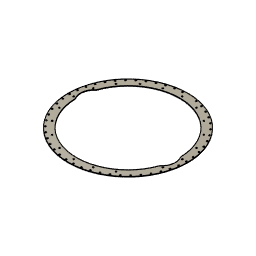
chopper_wheel v9 (Autodesk Fusion 360 design; units mm, degrees)
Autodesk Fusion 360 part; units mm, degrees
sketch "Sketch1" plane through (0, 0, 0) normal (0, 0, 1) x (1, 0, 0)
  circle A0 centre (0, 0) radius 190
  circle A1 centre (0, 0) radius 210
  dimension "d1" = 380
  dimension "d2" = 420
  constraint coincident A0.centre A1.centre
  constraint concentric A0 A1
  measures "d1" diameter of A0
  measures "d2" diameter of A1
extrude "Extrude1" add sketch "Sketch1" along normal blind 2
sketch "Sketch2" plane through (0, 0, 2) normal (0, 0, 1) x (-1, 0, 0)
  circle A0 centre (0, 0) radius 190
  circle A1 centre (0, 0) radius 210
  line L0 (200, 0) -> (190.2113, 61.8034)
  line L1 (190.2113, 61.8034) -> (161.8034, 117.5571)
  line L2 (161.8034, 117.5571) -> (117.5571, 161.8034)
  line L3 (117.5571, 161.8034) -> (61.8034, 190.2113)
  line L4 (61.8034, 190.2113) -> (0, 200)
  line L5 (0, 200) -> (-61.8034, 190.2113)
  line L6 (-61.8034, 190.2113) -> (-117.5571, 161.8034)
  line L7 (-117.5571, 161.8034) -> (-161.8034, 117.5571)
  line L8 (-161.8034, 117.5571) -> (-190.2113, 61.8034)
  line L9 (-190.2113, 61.8034) -> (-200, 0)
  line L10 (-200, 0) -> (-190.2113, -61.8034)
  line L11 (-190.2113, -61.8034) -> (-161.8034, -117.5571)
  line L12 (-161.8034, -117.5571) -> (-117.5571, -161.8034)
  line L13 (-117.5571, -161.8034) -> (-61.8034, -190.2113)
  line L14 (-61.8034, -190.2113) -> (0, -200)
  line L15 (0, -200) -> (61.8034, -190.2113)
  line L16 (61.8034, -190.2113) -> (117.5571, -161.8034)
  line L17 (117.5571, -161.8034) -> (161.8034, -117.5571)
  line L18 (161.8034, -117.5571) -> (190.2113, -61.8034)
  line L19 (190.2113, -61.8034) -> (200, 0)
  constraint coincident A0.centre A1.centre
hole "Hole1" at (-200, 0, 2) at (-190.2113, 61.8034, 2) at (-161.8034, 117.5571, 2) at (-117.5571, 161.8034, 2) at (-61.8034, 190.2113, 2) at (0, 200, 2) at (61.8034, 190.2113, 2) at (117.5571, 161.8034, 2) at (161.8034, 117.5571, 2) at (190.2113, 61.8034, 2) at (200, 0, 2) at (190.2113, -61.8034, 2) at (117.5571, -161.8034, 2) at (61.8034, -190.2113, 2) at (0, -200, 2) at (-61.8034, -190.2113, 2) at (-117.5571, -161.8034, 2) at (-161.8034, -117.5571, 2) at (-190.2113, -61.8034, 2) direction (0, 0, -1) diameter 4.5 depth 20 tip angle 180
sketch "Sketch3" plane through (0, 0, 2) normal (0, 0, 1) x (-1, 0, 0)
  circle A0 centre (161.8034, 117.5571) radius 2.25
  circle A1 centre (61.8034, 190.2113) radius 2.25
  circle A2 centre (-61.8034, 190.2113) radius 2.25
  circle A3 centre (-190.2113, 61.8034) radius 2.25
  circle A4 centre (-190.2113, -61.8034) radius 2.25
  circle A5 centre (-117.5571, -161.8034) radius 2.25
  circle A6 centre (0, -200) radius 2.25
  circle A7 centre (117.5571, -161.8034) radius 2.25
  circle A8 centre (190.2113, -61.8034) radius 2.25
  circle A9 centre (200, 0) radius 2.25
  circle A10 centre (161.8034, -117.5571) radius 2.25
  circle A11 centre (61.8034, -190.2113) radius 2.25
  circle A12 centre (-61.8034, -190.2113) radius 2.25
  circle A13 centre (-161.8034, -117.5571) radius 2.25
  circle A14 centre (-200, 0) radius 2.25
  circle A15 centre (-117.5571, 161.8034) radius 2.25
  circle A16 centre (0, 200) radius 2.25
  circle A17 centre (117.5571, 161.8034) radius 2.25
  circle A18 centre (190.2113, 61.8034) radius 2.25
  circle A19 centre (0, 0) radius 190
  circle A20 centre (0, 0) radius 210
  circle A21 centre (0, 0) radius 200
  line L0 (0, 0) -> (190.2113, -61.8034)
  line L1 (0, 0) -> (200, 0)
  line L2 (0, 0) -> (197.5377, -31.2869)
  line L3 (197.5377, -31.2869) -> (148.1533, -23.4652)
  circle A22 centre (148.1533, -23.4652) radius 50
  line L4 (197.5377, -31.2869) -> (-197.5377, 31.2869)
  line L5 (-197.5377, 31.2869) -> (-148.1533, 23.4652)
  circle A23 centre (-148.1533, 23.4652) radius 50
  dimension "d8" = 171
  dimension "d9" = 50
  dimension "d10" = 100
  dimension "d11" = 50
  dimension "d12" = 100
  constraint coincident A19.centre A20.centre
  constraint coincident A9.centre A21
  constraint coincident A8.centre L0.end
  constraint coincident A9.centre L1.end
  constraint parallel L2 L3
  constraint coincident L3.end A22.centre
  constraint coincident A21 L4.end
  constraint parallel L2 L4
  constraint coincident L4 L5.end
  constraint coincident L5.end A23.centre
  measures "d8" angle of L1 L2
  measures "d9" distance of L2.end L3.end
  measures "d10" diameter of A22
  measures "d11" distance of L4.end L5.end
  measures "d12" diameter of A23
extrude "Extrude2" cut sketch "Sketch3" against normal blind 2 contours A19 L1 L2 L3 A22 L4 | A19 L1 A22 | A19 L0 L2 L3 A22 L4 | A19 L0 A22 | A19 L4 L5 A23 | A19 L4 L5 A23 picked at (191.5682, -25.2216) picked at (191.2896, 0.4483) picked at (189.8761, -35.6021) picked at (181.7887, -59.5381) picked at (-189.6936, 36.3263) picked at (-191.6348, 24.0702)
sketch "Sketch4" plane through (0, 0, 2) normal (0, 0, 1) x (-1, 0, 0)
  arc A0 (179.4368, -62.4695) -> (189.9587, 3.9631) centre (148.1533, -23.4652) ccw
  arc A1 (-189.9587, -3.9631) -> (179.4368, -62.4695) centre (0, 0) ccw
  arc A2 (-179.4368, 62.4695) -> (-189.9587, -3.9631) centre (-148.1533, 23.4652) ccw
  arc A3 (189.9587, 3.9631) -> (-179.4368, 62.4695) centre (0, 0) ccw
  circle A4 centre (161.8034, 117.5571) radius 2.25
  circle A5 centre (61.8034, 190.2113) radius 2.25
  circle A6 centre (-61.8034, 190.2113) radius 2.25
  circle A7 centre (-190.2113, 61.8034) radius 2.25
  circle A8 centre (-190.2113, -61.8034) radius 2.25
  circle A9 centre (-117.5571, -161.8034) radius 2.25
  circle A10 centre (0, -200) radius 2.25
  circle A11 centre (117.5571, -161.8034) radius 2.25
  circle A12 centre (190.2113, -61.8034) radius 2.25
  circle A13 centre (200, 0) radius 2.25
  circle A14 centre (161.8034, -117.5571) radius 2.25
  circle A15 centre (61.8034, -190.2113) radius 2.25
  circle A16 centre (-61.8034, -190.2113) radius 2.25
  circle A17 centre (-161.8034, -117.5571) radius 2.25
  circle A18 centre (-200, 0) radius 2.25
  circle A19 centre (-117.5571, 161.8034) radius 2.25
  circle A20 centre (0, 200) radius 2.25
  circle A21 centre (117.5571, 161.8034) radius 2.25
  circle A22 centre (190.2113, 61.8034) radius 2.25
sketch "Sketch5" plane through (0, 0, 2) normal (0, 0, 1) x (-1, 0, 0)
  circle A0 centre (0, 0) radius 210
  circle A1 centre (0, 0) radius 220
  line L0 (-215, 0) -> (-213.3047, -26.9466)
  line L1 (-213.3047, -26.9466) -> (-208.2454, -53.4683)
  line L2 (-208.2454, -53.4683) -> (-199.9019, -79.1468)
  line L3 (-199.9019, -79.1468) -> (-188.4059, -103.577)
  line L4 (-188.4059, -103.577) -> (-173.9387, -126.3738)
  line L5 (-173.9387, -126.3738) -> (-156.7283, -147.1776)
  line L6 (-156.7283, -147.1776) -> (-137.0462, -165.6603)
  line L7 (-137.0462, -165.6603) -> (-115.2028, -181.5305)
  line L8 (-115.2028, -181.5305) -> (-91.5425, -194.5378)
  line L9 (-91.5425, -194.5378) -> (-66.4387, -204.4772)
  line L10 (-66.4387, -204.4772) -> (-40.287, -211.1918)
  line L11 (-40.287, -211.1918) -> (-13.5, -214.5757)
  line L12 (-13.5, -214.5757) -> (13.5, -214.5757)
  line L13 (13.5, -214.5757) -> (40.287, -211.1918)
  line L14 (40.287, -211.1918) -> (66.4387, -204.4772)
  line L15 (66.4387, -204.4772) -> (91.5425, -194.5378)
  line L16 (91.5425, -194.5378) -> (115.2028, -181.5305)
  line L17 (115.2028, -181.5305) -> (137.0462, -165.6603)
  line L18 (137.0462, -165.6603) -> (156.7283, -147.1776)
  line L19 (156.7283, -147.1776) -> (173.9387, -126.3738)
  line L20 (173.9387, -126.3738) -> (188.4059, -103.577)
  line L21 (188.4059, -103.577) -> (199.9019, -79.1468)
  line L22 (199.9019, -79.1468) -> (208.2454, -53.4683)
  line L23 (208.2454, -53.4683) -> (213.3047, -26.9466)
  line L24 (213.3047, -26.9466) -> (215, 0)
  line L25 (215, 0) -> (213.3047, 26.9466)
  line L26 (213.3047, 26.9466) -> (208.2454, 53.4683)
  line L27 (208.2454, 53.4683) -> (199.9019, 79.1468)
  line L28 (199.9019, 79.1468) -> (188.4059, 103.577)
  line L29 (188.4059, 103.577) -> (173.9387, 126.3738)
  line L30 (173.9387, 126.3738) -> (156.7283, 147.1776)
  line L31 (156.7283, 147.1776) -> (137.0462, 165.6603)
  line L32 (137.0462, 165.6603) -> (115.2028, 181.5305)
  line L33 (115.2028, 181.5305) -> (91.5425, 194.5378)
  line L34 (91.5425, 194.5378) -> (66.4387, 204.4772)
  line L35 (66.4387, 204.4772) -> (40.287, 211.1918)
  line L36 (40.287, 211.1918) -> (13.5, 214.5757)
  line L37 (13.5, 214.5757) -> (-13.5, 214.5757)
  line L38 (-13.5, 214.5757) -> (-40.287, 211.1918)
  line L39 (-40.287, 211.1918) -> (-66.4387, 204.4772)
  line L40 (-66.4387, 204.4772) -> (-91.5425, 194.5378)
  line L41 (-91.5425, 194.5378) -> (-115.2028, 181.5305)
  line L42 (-115.2028, 181.5305) -> (-137.0462, 165.6603)
  line L43 (-137.0462, 165.6603) -> (-156.7283, 147.1776)
  line L44 (-156.7283, 147.1776) -> (-173.9387, 126.3738)
  line L45 (-173.9387, 126.3738) -> (-188.4059, 103.577)
  line L46 (-188.4059, 103.577) -> (-199.9019, 79.1468)
  line L47 (-199.9019, 79.1468) -> (-208.2454, 53.4683)
  line L48 (-208.2454, 53.4683) -> (-213.3047, 26.9466)
  line L49 (-213.3047, 26.9466) -> (-215, 0)
  circle A2 centre (-215, 0) radius 2.5
  circle A3 centre (-213.3047, 26.9466) radius 2.5
  circle A4 centre (-208.2454, 53.4683) radius 2.5
  circle A5 centre (-199.9019, 79.1468) radius 2.5
  circle A6 centre (-188.4059, 103.577) radius 2.5
  circle A7 centre (-173.9387, 126.3738) radius 2.5
  circle A8 centre (-156.7283, 147.1776) radius 2.5
  circle A9 centre (-137.0462, 165.6603) radius 2.5
  circle A10 centre (-115.2028, 181.5305) radius 2.5
  circle A11 centre (-91.5425, 194.5378) radius 2.5
  circle A12 centre (-66.4387, 204.4772) radius 2.5
  circle A13 centre (-40.287, 211.1918) radius 2.5
  circle A14 centre (-13.5, 214.5757) radius 2.5
  circle A15 centre (13.5, 214.5757) radius 2.5
  circle A16 centre (40.287, 211.1918) radius 2.5
  circle A17 centre (66.4387, 204.4772) radius 2.5
  circle A18 centre (91.5425, 194.5378) radius 2.5
  circle A19 centre (115.2028, 181.5305) radius 2.5
  circle A20 centre (137.0462, 165.6603) radius 2.5
  circle A21 centre (156.7283, 147.1776) radius 2.5
  circle A22 centre (173.9387, 126.3738) radius 2.5
  circle A23 centre (188.4059, 103.577) radius 2.5
  circle A24 centre (199.9019, 79.1468) radius 2.5
  circle A25 centre (208.2454, 53.4683) radius 2.5
  circle A26 centre (213.3047, 26.9466) radius 2.5
  circle A27 centre (215, 0) radius 2.5
  circle A28 centre (213.3047, -26.9466) radius 2.5
  circle A29 centre (208.2454, -53.4683) radius 2.5
  circle A30 centre (199.9019, -79.1468) radius 2.5
  circle A31 centre (188.4059, -103.577) radius 2.5
  circle A32 centre (173.9387, -126.3738) radius 2.5
  circle A33 centre (156.7283, -147.1776) radius 2.5
  circle A34 centre (137.0462, -165.6603) radius 2.5
  circle A35 centre (115.2028, -181.5305) radius 2.5
  circle A36 centre (91.5425, -194.5378) radius 2.5
  circle A37 centre (66.4387, -204.4772) radius 2.5
  circle A38 centre (40.287, -211.1918) radius 2.5
  circle A39 centre (13.5, -214.5757) radius 2.5
  circle A40 centre (-13.5, -214.5757) radius 2.5
  circle A41 centre (-40.287, -211.1918) radius 2.5
  circle A42 centre (-66.4387, -204.4772) radius 2.5
  circle A43 centre (-91.5425, -194.5378) radius 2.5
  circle A44 centre (-115.2028, -181.5305) radius 2.5
  circle A45 centre (-137.0462, -165.6603) radius 2.5
  circle A46 centre (-156.7283, -147.1776) radius 2.5
  circle A47 centre (-173.9387, -126.3738) radius 2.5
  circle A48 centre (-188.4059, -103.577) radius 2.5
  circle A49 centre (-213.3047, -26.9466) radius 2.5
  circle A50 centre (-208.2454, -53.4683) radius 2.5
  circle A51 centre (-199.9019, -79.1468) radius 2.5
  dimension "d15" = 420
  dimension "d16" = 440
  dimension "d17" = 215
  dimension "d18" = 5
  dimension "d19" = 5
  dimension "d20" = 5
  dimension "d21" = 5
  dimension "d22" = 5
  dimension "d23" = 5
  dimension "d24" = 5
  dimension "d25" = 5
  dimension "d26" = 5
  dimension "d27" = 5
  dimension "d28" = 5
  dimension "d29" = 5
  dimension "d30" = 5
  dimension "d31" = 5
  dimension "d32" = 5
  dimension "d33" = 5
  dimension "d34" = 5
  dimension "d35" = 5
  dimension "d36" = 5
  dimension "d37" = 5
  dimension "d38" = 5
  dimension "d39" = 5
  dimension "d40" = 5
  dimension "d41" = 5
  dimension "d42" = 5
  dimension "d43" = 5
  dimension "d44" = 5
  dimension "d45" = 5
  dimension "d46" = 5
  dimension "d47" = 5
  dimension "d48" = 5
  dimension "d49" = 5
  dimension "d50" = 5
  dimension "d51" = 5
  dimension "d52" = 5
  dimension "d53" = 5
  dimension "d54" = 5
  dimension "d55" = 5
  dimension "d56" = 5
  dimension "d57" = 5
  dimension "d58" = 5
  dimension "d59" = 5
  dimension "d60" = 5
  dimension "d61" = 5
  dimension "d62" = 5
  dimension "d63" = 5
  dimension "d64" = 5
  dimension "d65" = 5
  dimension "d66" = 5
  dimension "d67" = 5
  constraint coincident A0.centre A1.centre
  constraint concentric A0 A1
  constraint coincident L0.start L49.end
  constraint coincident L48.end L49.start
  constraint coincident L47.end L48.start
  constraint coincident L46.end L47.start
  constraint coincident L45.end L46.start
  constraint coincident L44.end L45.start
  constraint coincident L43.end L44.start
  constraint coincident L42.end L43.start
  constraint coincident L41.end L42.start
  constraint coincident L40.end L41.start
  constraint coincident L39.end L40.start
  constraint coincident L38.end L39.start
  constraint coincident L37.end L38.start
  constraint coincident L36.end L37.start
  constraint coincident L35.end L36.start
  constraint coincident L34.end L35.start
  constraint coincident L33.end L34.start
  constraint coincident L32.end L33.start
  constraint coincident L31.end L32.start
  constraint coincident L30.end L31.start
  constraint coincident L29.end L30.start
  constraint coincident L28.end L29.start
  constraint coincident L27.end L28.start
  constraint coincident L26.end L27.start
  constraint coincident L25.end L26.start
  constraint coincident L24.end L25.start
  constraint coincident L23.end L24.start
  constraint coincident L22.end L23.start
  constraint coincident L21.end L22.start
  constraint coincident L20.end L21.start
  constraint coincident L19.end L20.start
  constraint coincident L18.end L19.start
  constraint coincident L17.end L18.start
  constraint coincident L16.end L17.start
  constraint coincident L15.end L16.start
  constraint coincident L14.end L15.start
  constraint coincident L13.end L14.start
  constraint coincident L12.end L13.start
  constraint coincident L11.end L12.start
  constraint coincident L10.end L11.start
  constraint coincident L9.end L10.start
  constraint coincident L8.end L9.start
  constraint coincident L7.end L8.start
  constraint coincident L6.end L7.start
  constraint coincident L5.end L6.start
  constraint coincident L4.end L5.start
  constraint coincident L3.end L4.start
  constraint coincident L0.end L1.start
  constraint coincident L1.end L2.start
  constraint coincident L2.end L3.start
  measures "d15" diameter of A0
  measures "d16" diameter of A1
  measures "d17" distance of L0.start A0.centre
  measures "d18" diameter of A2
  measures "d19" diameter of A3
  measures "d20" diameter of A4
  measures "d21" diameter of A5
  measures "d22" diameter of A6
  measures "d23" diameter of A7
  measures "d24" diameter of A8
  measures "d25" diameter of A9
  measures "d26" diameter of A10
  measures "d27" diameter of A11
  measures "d28" diameter of A12
  measures "d29" diameter of A13
  measures "d30" diameter of A14
  measures "d31" diameter of A15
  measures "d32" diameter of A16
  measures "d33" diameter of A17
  measures "d34" diameter of A18
  measures "d35" diameter of A19
  measures "d36" diameter of A20
  measures "d37" diameter of A21
  measures "d38" diameter of A22
  measures "d39" diameter of A23
  measures "d40" diameter of A24
  measures "d41" diameter of A25
  measures "d42" diameter of A26
  measures "d43" diameter of A27
  measures "d44" diameter of A28
  measures "d45" diameter of A29
  measures "d46" diameter of A30
  measures "d47" diameter of A31
  measures "d48" diameter of A32
  measures "d49" diameter of A33
  measures "d50" diameter of A34
  measures "d51" diameter of A35
  measures "d52" diameter of A36
  measures "d53" diameter of A37
  measures "d54" diameter of A38
  measures "d55" diameter of A39
  measures "d56" diameter of A40
  measures "d57" diameter of A41
  measures "d58" diameter of A42
  measures "d59" diameter of A43
  measures "d60" diameter of A44
  measures "d61" diameter of A45
  measures "d62" diameter of A46
  measures "d63" diameter of A47
  measures "d64" diameter of A48
  measures "d65" diameter of A49
  measures "d66" diameter of A50
  measures "d67" diameter of A51
extrude "Extrude3" add sketch "Sketch5" against normal blind 2 contours A1 | L0 L1 L2 L3 L4 L5 L6 L7 L8 L9 L10 L11 L12 L13 L14 L15 L16 L17 L18 L19 L20 L21 L22 L23 L24 L25 L26 L27 L28 L29 L30 L31 L32 L33 L34 L35 L36 L37 L38 L39 L40 L41 L42 L43 L44 L45 L46 L47 L48 L49 A2 A3 A4 A5 A6 A7 A8 A9 A10 A11 A12 A13 A14 A15 A16 A17 A18 A19 A20 A21 A22 A23 A24 A25 A26 A27 A28 A29 A30 A31 A32 A33 A34 A35 A36 A37 A38 A39 A40 A41 A42 A43 A44 A45 A46 A47 A48 A49 A50 A51
sketch "Sketch6" plane through (0, 0, 2) normal (0, 0, 1) x (-1, 0, 0)
  circle A0 centre (0, 0) radius 220
  circle A1 centre (188.4059, 103.577) radius 2.5
  circle A2 centre (-137.0462, 165.6603) radius 2.5
  circle A3 centre (91.5425, 194.5378) radius 2.5
  circle A4 centre (-66.4387, 204.4772) radius 2.5
  circle A5 centre (66.4387, 204.4772) radius 2.5
  circle A6 centre (173.9387, 126.3738) radius 2.5
  circle A7 centre (115.2028, -181.5305) radius 2.5
  circle A8 centre (199.9019, -79.1468) radius 2.5
  circle A9 centre (40.287, -211.1918) radius 2.5
  circle A10 centre (156.7283, 147.1776) radius 2.5
  circle A11 centre (-13.5, 214.5757) radius 2.5
  circle A12 centre (-40.287, 211.1918) radius 2.5
  circle A13 centre (137.0462, 165.6603) radius 2.5
  circle A14 centre (213.3047, -26.9466) radius 2.5
  circle A15 centre (213.3047, 26.9466) radius 2.5
  circle A16 centre (215, 0) radius 2.5
  circle A17 centre (208.2454, -53.4683) radius 2.5
  circle A18 centre (13.5, 214.5757) radius 2.5
  circle A19 centre (156.7283, -147.1776) radius 2.5
  circle A20 centre (115.2028, 181.5305) radius 2.5
  circle A21 centre (91.5425, -194.5378) radius 2.5
  circle A22 centre (199.9019, 79.1468) radius 2.5
  circle A23 centre (66.4387, -204.4772) radius 2.5
  circle A24 centre (137.0462, -165.6603) radius 2.5
  circle A25 centre (-115.2028, 181.5305) radius 2.5
  circle A26 centre (173.9387, -126.3738) radius 2.5
  circle A27 centre (-91.5425, 194.5378) radius 2.5
  circle A28 centre (208.2454, 53.4683) radius 2.5
  circle A29 centre (188.4059, -103.577) radius 2.5
  circle A30 centre (40.287, 211.1918) radius 2.5
  circle A31 centre (-13.5, -214.5757) radius 2.5
  circle A32 centre (-91.5425, -194.5378) radius 2.5
  circle A33 centre (-173.9387, 126.3738) radius 2.5
  circle A34 centre (-188.4059, 103.577) radius 2.5
  circle A35 centre (-199.9019, 79.1468) radius 2.5
  circle A36 centre (-208.2454, 53.4683) radius 2.5
  circle A37 centre (-213.3047, 26.9466) radius 2.5
  circle A38 centre (-215, 0) radius 2.5
  circle A39 centre (-213.3047, -26.9466) radius 2.5
  circle A40 centre (-208.2454, -53.4683) radius 2.5
  circle A41 centre (-199.9019, -79.1468) radius 2.5
  circle A42 centre (-188.4059, -103.577) radius 2.5
  circle A43 centre (-173.9387, -126.3738) radius 2.5
  circle A44 centre (-156.7283, -147.1776) radius 2.5
  circle A45 centre (-137.0462, -165.6603) radius 2.5
  circle A46 centre (-115.2028, -181.5305) radius 2.5
  circle A47 centre (-40.287, -211.1918) radius 2.5
  circle A48 centre (13.5, -214.5757) radius 2.5
  circle A49 centre (-66.4387, -204.4772) radius 2.5
  circle A50 centre (-156.7283, 147.1776) radius 2.5
  arc A51 (179.4368, -62.4695) -> (189.9587, 3.9631) centre (148.1533, -23.4652) ccw
  arc A52 (-189.9587, -3.9631) -> (179.4368, -62.4695) centre (0, 0) ccw
  arc A53 (-179.4368, 62.4695) -> (-189.9587, -3.9631) centre (-148.1533, 23.4652) ccw
  arc A54 (189.9587, 3.9631) -> (-179.4368, 62.4695) centre (0, 0) ccw
  circle A55 centre (161.8034, 117.5571) radius 2.25
  circle A56 centre (61.8034, 190.2113) radius 2.25
  circle A57 centre (-61.8034, 190.2113) radius 2.25
  circle A58 centre (-190.2113, 61.8034) radius 2.25
  circle A59 centre (-190.2113, -61.8034) radius 2.25
  circle A60 centre (-117.5571, -161.8034) radius 2.25
  circle A61 centre (0, -200) radius 2.25
  circle A62 centre (117.5571, -161.8034) radius 2.25
  circle A63 centre (190.2113, -61.8034) radius 2.25
  circle A64 centre (200, 0) radius 2.25
  circle A65 centre (161.8034, -117.5571) radius 2.25
  circle A66 centre (61.8034, -190.2113) radius 2.25
  circle A67 centre (-61.8034, -190.2113) radius 2.25
  circle A68 centre (-161.8034, -117.5571) radius 2.25
  circle A69 centre (-200, 0) radius 2.25
  circle A70 centre (-117.5571, 161.8034) radius 2.25
  circle A71 centre (0, 200) radius 2.25
  circle A72 centre (117.5571, 161.8034) radius 2.25
  circle A73 centre (190.2113, 61.8034) radius 2.25
  circle A74 centre (-13.5, -214.5757) radius 2.5
  constraint concentric A31 A74
extrude "Extrude4" add sketch "Sketch6" against normal blind 2 contours A31 A74
